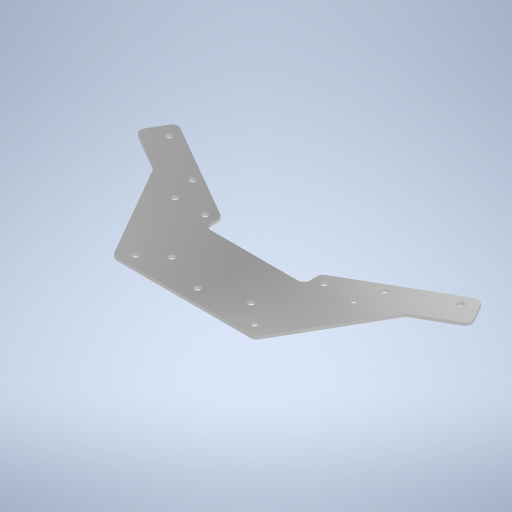
# Autodesk Inventor part: upper_plate
Saved by Autodesk Inventor 2024.1 (Build 281209000, 209)
## iProperties
Created: 2025-02-03
Part Number: upper_plate
Material: アルミニウム 6061
Document SubType Name: Sheet Metal
Designer: hibik
Density: 2.7 g/cm^3
Sheet Metal Rule: Default_mm
Appearance: アルミニウム - フラット
Author: hibik
Autodesk Inventor part; units mm, degrees
ref_plane "YZ Plane" through (0, 0, 0) normal (1, 0, 0) x (0, 1, 0)
ref_plane "XZ Plane" through (0, 0, 0) normal (0, 1, 0) x (-1, 0, 0)
ref_plane "XY Plane" through (0, 0, 0) normal (0, 0, 1) x (1, 0, 0)
sketch "スケッチ1" plane through (0, 0, 0) normal (0, 1, 0) x (-1, 0, 0)
  line L0 (75, 0) -> (105, -51.9615)
  line L1 (-75, 0) -> (-105, -51.9615)
  line L2 (0, -218.2384) -> (0, 36.3731)
  line L3 (147, 0) -> (-147, 0)
  line L4 (105, -51.9615) -> (30, -181.8653)
  line L5 (30, -181.8653) -> (-30, -181.8653)
  line L6 (-30, -181.8653) -> (-105, -51.9615)
  line L7 (75, 0) -> (-75, 0)
  line L8 (34, 0) -> (34, -24.3509)
  line L9 (34, -24.3509) -> (48.7058, -49.822)
  line L10 (48.7058, -49.822) -> (90, -25.9808)
  line L11 (45, 0) -> (45, -18) construction
  line L12 (45, -18) -> (34, -24.3509) construction
  line L13 (84.5, -87.4686) -> (63.4115, -75.2931)
  line L14 (63.4115, -75.2931) -> (48.7058, -49.822)
  line L15 (-34, 0) -> (-34, -24.3509)
  line L16 (-34, -24.3509) -> (-48.7058, -49.822)
  line L17 (-63.4115, -75.2931) -> (-48.7058, -49.822)
  line L18 (-84.5, -87.4686) -> (-63.4115, -75.2931)
  circle A0 centre (30, -32.75) radius 1.6
  circle A1 centre (-30, -32.75) radius 1.6
  line L19 (35.5295, -27) -> (-35.5295, -27)
  point P0 (0, 0)
  point P1 (0, 0)
  point P2 (0, -27)
  dimension "d1" = 150
  dimension "d2" = 60
  dimension "d3" = 60
  dimension "d6" = 60
  dimension "d30" = 60
  dimension "d31" = 18
  dimension "d32" = 30
  dimension "d33" = 41
  dimension "d34" = 3.2
  dimension "d35" = 30
  dimension "d36" = 32.75
  dimension "d37" = 27
  measures "d1" distance of L1.start L0.start
  measures "d2" angle of L3 L0
  measures "d3" angle of L1 L3
  measures "d6" distance of L4.end L5.end
  measures "d30" angle of L11 L12
  measures "d31" distance of L11.start L11.end
  measures "d32" distance of L0.start L11.start
  measures "d33" distance of L0.start L8.start
  measures "d34" diameter of A0
  measures "d35" distance from line of L2 A0.centre
  measures "d36" distance from line of L7 A0.centre
  measures "d37" distance between parallel lines of L7 L19
extrude "プレート1" add sketch "スケッチ1" along normal blind 1.5 contours L14 L13 L4 L5 L2 L19 L9 | L2 L5 L6 L18 L17 L16 L19
sketch "スケッチ4" plane through (0, 1.5, 0) normal (0, 1, 0) x (1, 0, 0)
  circle A0 centre (30, 67.8013) radius 1.6
  circle A1 centre (45, 67.8013) radius 1.6
  line L0 (0, 218.2384) -> (0, -36.3731)
  circle A2 centre (-30, 67.8013) radius 1.6
  circle A3 centre (-45, 67.8013) radius 1.6
  line L1 (61.6173, 73.1025) -> (25, 73.1025) construction
  line L2 (25, 73.1025) -> (25, 62.5) construction
  line L3 (-61.6173, 73.1025) -> (-25, 73.1025) construction
  line L4 (-25, 73.1025) -> (-25, 62.5) construction
  line L5 (-25, 62.5) -> (25, 62.5)
  line L6 (30, 73.1025) -> (30, 181.8653)
  line L7 (30, 181.8653) -> (-30, 181.8653)
  line L8 (-30, 181.8653) -> (-30, 73.1025)
  line L9 (-25, 62.5) -> (25, 62.5)
  line L10 (25, 62.5) -> (25, 71.0141)
  line L11 (-25, 71.0141) -> (-25, 62.5)
  line L12 (30, 181.8653) -> (84.5, 87.4686)
  line L13 (76.75, 100.892) -> (30, 73.9008)
  line L14 (-30, 73.9008) -> (-76.75, 100.892)
  line L15 (-84.5, 87.4686) -> (-30, 181.8653)
  line L16 (84.5, 87.4686) -> (63.4115, 75.2931)
  line L17 (-63.4115, 75.2931) -> (-84.5, 87.4686)
  line L18 (-35.5295, 27) -> (-63.4115, 75.2931)
  line L19 (62.8673, 70.9375) -> (54.6673, 85.1403)
  arc A4 (54.6673, 85.1403) -> (44.275, 79.1403) centre (49.4712, 82.1403) ccw
  line L20 (44.275, 79.1403) -> (52.475, 64.9375)
  line L21 (52.475, 64.9375) -> (62.8673, 70.9375)
  line L22 (51.2321, 85.1903) -> (52.993, 82.1403)
  line L23 (52.993, 82.1403) -> (51.2321, 79.0903)
  line L24 (51.2321, 79.0903) -> (47.7102, 79.0903)
  line L25 (47.7102, 79.0903) -> (45.9493, 82.1403)
  line L26 (45.9493, 82.1403) -> (47.7102, 85.1903)
  line L27 (47.7102, 85.1903) -> (51.2321, 85.1903)
  line L28 (-30, 73.9008) -> (-25, 71.0141)
  line L29 (30, 73.9008) -> (25, 71.0141)
  point P0 (0, 0)
extrude "切り取り3" cut sketch "スケッチ4" against normal blind 1.5 contours A0 | A1 | L7 L6 L29 L10 L5 L0 | L0 L5 L11 L28 L8 L7 | L12 L13 A4 L6 | L8 L14 L15 | A4 L13 L27 L26 | L26 L27 L13 | A2 | A3
sketch "スケッチ5" plane through (0, 1.5, 0) normal (0, 1, 0) x (1, 0, 0)
  line L0 (-75, 44) -> (75, 44) projected
  circle A0 centre (-20, 41) radius 3
  circle A1 centre (20, 41) radius 3
  line L1 (-25, 62.5) -> (25, 62.5) projected
  line L2 (0, 62.5) -> (0, 27)
  line L3 (35.5295, 27) -> (-35.5295, 27) projected
  circle A2 centre (-20, 41) radius 1.6
  circle A3 centre (20, 41) radius 1.6
  circle A4 centre (0, 34) radius 1.6
  point P0 (0, 0)
  dimension "d41" = 6
  dimension "d42" = 6
  dimension "d43" = 40
  dimension "d44" = 3.2
  dimension "d45" = 3.2
  dimension "d46" = 3.2
  dimension "d47" = 7
  constraints: 5 centre point, 2 coincident, 2 end point, 2 midpoint, 1 point on line, 1 symmetric about line, 1 tangent
  measures "d41" diameter of A0
  measures "d42" diameter of A1
  measures "d43" distance of A1.centre A0.centre
  measures "d44" diameter of A2
  measures "d45" diameter of A3
  measures "d46" diameter of A4
  measures "d47" vertical distance of A0.centre A4.centre
extrude "切り取り4" cut sketch "スケッチ5" against normal blind 1.5 contours A4 L2 | L2 A4 | A2 | A3
sketch "スケッチ6" plane through (0, 1.5, 0) normal (0, 1, 0) x (1, 0, 0)
  ellipse E0 centre (-73.3666, 93.1522) end of major axis (-72.2841, 92.5272) minor radius 1.2133 projected
  circle A0 centre (-48.4391, 79.9279) radius 1.6
  circle A1 centre (-73.3666, 93.1522) radius 1.6
  line L0 (0, 0) -> (0, 20.4537)
  circle A2 centre (48.4391, 79.9279) radius 1.6
  circle A3 centre (73.3666, 93.1522) radius 1.6
  circle A4 centre (-48.4391, 79.9279) radius 1.35 projected
  dimension "d51" = 3.2
  dimension "d52" = 3.2
  constraints: 4 centre point, 2 end point, 2 symmetric about line, 1 coincident, 1 vertical, 2 other
  measures "d51" diameter of A0
  measures "d52" diameter of A1
extrude "切り取り5" cut sketch "スケッチ6" against normal blind 1.5 contours E0 | A0 | A1 | A2 | A3 | A4
fillet "フィレット2" radius 3 12 edges at (-84.5, 0.75, -87.4686) (-76.75, 0.75, -100.892) (-63.4115, 0.75, -75.2931) (-35.5295, 0.75, -27) (35.5295, 0.75, -27) (63.4115, 0.75, -75.2931) (84.5, 0.75, -87.4686) (76.75, 0.75, -100.892) (25, 0.75, -62.5) (-25, 0.75, -62.5) (-25, 0.75, -71.0141) (25, 0.75, -71.0141)
equation "\"d3\" = d2"
equation "\"d38\" = Thickness"
equation "\"d41\" = d42"
equation "\"d48\" = Thickness"
equation "\"d53\" = Thickness"
equation "\"d16\" = Thickness"
equation "\"BendRadius\" = Thickness"
equation "\"BendReliefWidth\" = Thickness"
equation "\"BendReliefDepth\" = 0.5 * Thickness"
equation "\"CornerReliefSize\" = 4 * Thickness"
equation "\"MinimumRemnant\" = 2 * Thickness"
equation "\"TransitionRadius\" = BendRadius"
equation "\"JacobiRadiusSize\" = BendRadius"
equation "\"GapSize\" = Thickness"
equation "\"Thickness\" = 1.5"
